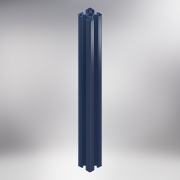
# Autodesk Inventor part: trail
Saved by Autodesk Inventor 2020 (Build 240168000, 168)
## iProperties
Created: 2017-06-26
Part Number: trail
Material: Aluminum 6061
Document SubType Name: Modeling
Designer: PC  USER
Density: 2.7 g/cm^3
Appearance: Flaked Satin - Blue
Author: PC  USER
Autodesk Inventor part; units mm, degrees
ref_plane "YZ Plane" through (0, 0, 0) normal (1, 0, 0) x (0, 1, 0)
ref_plane "XZ Plane" through (0, 0, 0) normal (0, 1, 0) x (-1, 0, 0)
ref_plane "XY Plane" through (0, 0, 0) normal (0, 0, 1) x (1, 0, 0)
sketch "Sketch1" plane through (0, 0, 0) normal (0, 0, 1) x (1, 0, 0)
  circle A0 centre (0, 0) radius 5
  arc A1 (-13, 15) -> (-15, 13) centre (-13, 13) ccw
  arc A2 (-15, -13) -> (-13, -15) centre (-13, -13) ccw
  arc A3 (13, -15) -> (15, -13) centre (13, -13) ccw
  arc A4 (15, 13) -> (13, 15) centre (13, 13) ccw
  arc A5 (-13, 14) -> (-14, 13) centre (-13, 13) ccw
  arc A6 (-14, -13) -> (-13, -14) centre (-13, -13) ccw
  arc A7 (13, -14) -> (14, -13) centre (13, -13) ccw
  arc A8 (14, 13) -> (13, 14) centre (13, 13) ccw
  line L0 (14, -14) -> (-14, 14) construction
  line L1 (-14, -14) -> (14, 14) construction
  line L2 (15, -15) -> (-15, 15) construction
  line L3 (-15, -15) -> (15, 15) construction
  line L4 (-13, 15) -> (-8, 15)
  line L5 (-8, 13) -> (-8, 8) construction
  line L6 (-9.4142, 8) -> (-13, 8)
  line L7 (-15, 8) -> (-15, 13)
  line L8 (-13, -15) -> (-8, -15)
  line L9 (-8, -13) -> (-8, -9.4142)
  line L10 (-9.4142, -8) -> (-13, -8)
  line L11 (-15, -8) -> (-15, -13)
  line L12 (13, -15) -> (8, -15)
  line L13 (8, -13) -> (8, -9.4142)
  line L14 (9.4142, -8) -> (13, -8)
  line L15 (15, -8) -> (15, -13)
  line L16 (13, 15) -> (8, 15)
  line L17 (8, 13) -> (8, 9.4142)
  line L18 (9.4142, 8) -> (13, 8)
  line L19 (15, 8) -> (15, 13)
  line L20 (-13, 9) -> (-10, 9)
  line L21 (-9, 10) -> (-9, 13)
  line L22 (-10, 14) -> (-13, 14)
  line L23 (-14, 13) -> (-14, 10)
  line L24 (13, 9) -> (10, 9)
  line L25 (9, 10) -> (9, 13)
  line L26 (10, 14) -> (13, 14)
  line L27 (14, 13) -> (14, 10)
  line L28 (13, -9) -> (10, -9)
  line L29 (9, -10) -> (9, -13)
  line L30 (10, -14) -> (13, -14)
  line L31 (14, -13) -> (14, -10)
  line L32 (-13, -9) -> (-10, -9)
  line L33 (-9, -10) -> (-9, -13)
  line L34 (-10, -14) -> (-13, -14)
  line L35 (-14, -13) -> (-14, -10)
  line L36 (-14, 13) -> (-14, 10)
  line L37 (-14, -10) -> (-14, -13)
  line L38 (-14, -13) -> (-14, -10)
  line L39 (-14, 10) -> (-14, 13)
  line L40 (13, -15) -> (5, -15)
  line L41 (-5, -15) -> (-13, -15)
  line L42 (13, -15) -> (5, -15) construction
  line L43 (0, -15) -> (-13, -15) construction
  line L44 (4, -13) -> (8, -13)
  line L45 (-8, -13) -> (-4, -13)
  line L46 (10, -9) -> (13, -9)
  line L47 (14, -10) -> (14, -13)
  line L48 (13, -14) -> (10, -14)
  line L49 (9, -13) -> (9, -10)
  line L50 (5, -14) -> (5, -15)
  line L51 (13, -14) -> (10, -14)
  line L52 (5, -14) -> (4, -14)
  line L53 (4, -14) -> (5, -14)
  line L54 (10, -14) -> (13, -14)
  line L55 (-4, -14) -> (-5, -14)
  line L56 (-10, -14) -> (-13, -14)
  line L57 (-13, -14) -> (-10, -14)
  line L58 (-5, -14) -> (-4, -14)
  line L59 (14, -13) -> (14, -10)
  line L60 (14, 10) -> (14, 13)
  line L61 (14, 13) -> (14, 10)
  line L62 (14, -10) -> (14, -13)
  line L63 (-5, -14) -> (-5, -15)
  line L64 (10, 14) -> (13, 14)
  line L65 (13, 14) -> (10, 14)
  line L66 (-10, 14) -> (-13, 14)
  line L67 (-13, 14) -> (-10, 14)
  line L68 (-5, 15) -> (-5, 14)
  line L69 (-13, 15) -> (-5, 15)
  line L70 (5, 15) -> (13, 15)
  line L71 (-15, 15) -> (-5, 15) construction
  line L72 (5, 15) -> (15, 15) construction
  line L73 (5, 15) -> (5, 14)
  line L74 (8, 13) -> (4, 13)
  line L75 (5, 14) -> (4, 14)
  line L76 (-5, 14) -> (-4, 14)
  line L77 (4, 14) -> (5, 14)
  line L78 (-4, 13) -> (-8, 13)
  line L79 (-4, 14) -> (-5, 14)
  line L80 (4, 13) -> (4, 14)
  line L81 (-4, 13) -> (-4, 14)
  line L82 (-4, -14) -> (-4, -13)
  line L83 (4, -14) -> (4, -13)
  line L84 (-8, 9.4142) -> (-4.1919, 5.6061)
  line L85 (8, 9.4142) -> (4.1919, 5.6061)
  line L86 (9.4142, 8) -> (5.6061, 4.1919)
  line L87 (5.6061, -4.1919) -> (9.4142, -8)
  line L88 (4.1919, -5.6061) -> (8, -9.4142)
  line L89 (-4.1919, -5.6061) -> (-8, -9.4142)
  line L90 (-5.6061, -4.1919) -> (-9.4142, -8)
  line L91 (-9.4142, 8) -> (-5.6061, 4.1919)
  arc A9 (4.1919, 5.6061) -> (-4.1919, 5.6061) centre (0, 0) ccw
  arc A10 (5.6061, -4.1919) -> (5.6061, 4.1919) centre (0, 0) ccw
  arc A11 (-5.6061, 4.1919) -> (-5.6061, -4.1919) centre (0, 0) ccw
  arc A12 (-4.1919, -5.6061) -> (4.1919, -5.6061) centre (0, 0) ccw
  line L92 (-8, 13) -> (-8, 9.4142)
  line L93 (-15, -13) -> (-15, -5) construction
  line L94 (-15, -13) -> (-15, -5)
  line L95 (-15, 5) -> (-15, 13)
  line L96 (15, -5) -> (15, -13) construction
  line L97 (15, 13) -> (15, 5)
  line L98 (15, -5) -> (15, -13)
  line L99 (-14, -4) -> (-14, -5)
  line L100 (14, -4) -> (14, -5)
  line L101 (14, 4) -> (14, 5)
  line L102 (-14, 4) -> (-14, 5)
  line L103 (-13, 8) -> (-13, 4)
  line L104 (13, 4) -> (13, 8)
  line L105 (13, -8) -> (13, -4)
  line L106 (-13, -4) -> (-13, -8)
  line L107 (-14, -5) -> (-15, -5)
  line L108 (15, -5) -> (14, -5)
  line L109 (15, 5) -> (14, 5)
  line L110 (-14, 5) -> (-15, 5)
  line L111 (13, 4) -> (14, 4)
  line L112 (-14, 4) -> (-13, 4)
  line L113 (-14, -4) -> (-13, -4)
  line L114 (13, -4) -> (14, -4)
  arc A13 (-13, -9) -> (-14, -10) centre (-13, -10) ccw
  arc A14 (-9, -10) -> (-10, -9) centre (-10, -10) ccw
  arc A15 (-10, -14) -> (-9, -13) centre (-10, -13) ccw
  arc A16 (10, -9) -> (9, -10) centre (10, -10) ccw
  arc A17 (9, -13) -> (10, -14) centre (10, -13) ccw
  arc A18 (14, -10) -> (13, -9) centre (13, -10) ccw
  arc A19 (10, 14) -> (9, 13) centre (10, 13) ccw
  arc A20 (9, 10) -> (10, 9) centre (10, 10) ccw
  arc A21 (13, 9) -> (14, 10) centre (13, 10) ccw
  arc A22 (-9, 13) -> (-10, 14) centre (-10, 13) ccw
  arc A23 (-10, 9) -> (-9, 10) centre (-10, 10) ccw
  arc A24 (-14, 10) -> (-13, 9) centre (-13, 10) ccw
  point P0 (15, -15)
  point P1 (-5.5858, -7)
  dimension "d0" = 30
  dimension "d1" = 30
  dimension "d2" = 10
  dimension "d4" = 2
  dimension "d11" = 28
  dimension "d12" = 7
  dimension "d13" = 7
  dimension "d15" = 1
  dimension "d16" = 1
  dimension "d17" = 1
  dimension "d18" = 1
  dimension "d19" = 5
  dimension "d23" = 30
  dimension "d27" = 1
  dimension "d30" = 3.5858
  dimension "d31" = 2
  dimension "d32" = 16
  dimension "d33" = 8
  dimension "d34" = 6
  dimension "d35" = 5.5858
  constraints: 230 end point, 79 parallel, 48 point on circle, 40 tangent, 39 perpendicular, 25 centre point, 14 equal radius, 13 horizontal, 5 point on line, 4 midpoint, 1 coincident, 1 collinear
  measures "d0" distance of L2.end point (15, 15)
  measures "d1" distance of point (15, 15) point (15, -15)
  measures "d2" diameter of A0
  measures "d4" radius of A1
  measures "d11" distance of L0.end L1.end
  measures "d12" distance of L5.end L7.start
  measures "d13" distance of L4.end L5.end
  measures "d15" distance between parallel lines of L6 L20
  measures "d16" distance between parallel lines of L18 L24
  measures "d17" distance between parallel lines of L14 L28
  measures "d18" distance between parallel lines of L10 L32
  measures "d19" distance of L40.end L43.start
  measures "d23" distance of L93.end L96.start
  measures "d27" radius of A13
  measures "d30" distance of L13.start L13.end
  measures "d31" distance between parallel lines of L44 L40
  measures "d32" distance between parallel lines of L9 L13
  measures "d33" distance between parallel lines of L82 L83
  measures "d34" distance edge to line of A12 L44
  measures "d35" horizontal distance of A0.centre point (-5.586, -7)
extrude "Extrusion1" add sketch "Sketch1" along normal mid plane 318
equation "\"d1\" = d0"
body "Solid1"
